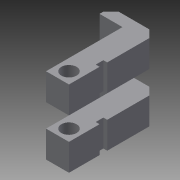
# Autodesk Inventor part: arms01
Saved by Autodesk Inventor 2015 (Build 190159000, 159)
## iProperties
Created: 2016-09-16
Part Number: arms01
Material: Generic
Document SubType Name: Modeling
Designer: spichelh
Density: 1 g/cm^3
Appearance: Default
Author: spichelh
Autodesk Inventor part; units mm, degrees
ref_plane "YZ Plane" through (0, 0, 0) normal (1, 0, 0) x (0, 1, 0)
ref_plane "XZ Plane" through (0, 0, 0) normal (0, 1, 0) x (-1, 0, 0)
ref_plane "XY Plane" through (0, 0, 0) normal (0, 0, 1) x (1, 0, 0)
sketch "Sketch1" plane through (0, 0, 0) normal (0, 0, 1) x (1, 0, 0)
  line L0 (16.7529, 22.7773) -> (28.7529, 22.7773)
  line L1 (28.7529, 22.7773) -> (28.7529, 15.7773)
  line L2 (28.7529, 15.7773) -> (16.7529, 15.7773)
  line L3 (16.7529, 15.7773) -> (16.7529, 22.7773)
  line L4 (16.7529, 9.7773) -> (28.7529, 9.7773)
  line L5 (28.7529, 9.7773) -> (28.7529, 2.7773)
  line L6 (28.7529, 2.7773) -> (16.7529, 2.7773)
  line L7 (16.7529, 2.7773) -> (16.7529, 9.7773)
  point P0 (0, 0)
  dimension "d0" = 7
  dimension "d1" = 6
  dimension "d2" = 12
  constraints: 16 end point, 4 parallel, 2 collinear, 2 horizontal, 2 perpendicular, 1 point on line
  measures "d0" distance of L6.end L4.start
  measures "d1" distance between parallel lines of L2 L4
  measures "d2" distance between parallel lines of L1 L3
extrude "Extrusion1" add sketch "Sketch1" along normal blind 3
sketch "Sketch2" plane through (0, 0, 3) normal (0, 0, 1) x (1, 0, 0)
  line L0 (16.7529, 15.7773) -> (28.7529, 15.7773) projected
  line L1 (28.7529, 22.7773) -> (22.7529, 22.7773)
  line L2 (22.7529, 22.7773) -> (22.7529, 15.7773)
  line L3 (22.7529, 15.7773) -> (28.7529, 15.7773)
  line L4 (28.7529, 15.7773) -> (28.7529, 22.7773)
  line L5 (28.7529, 22.7773) -> (16.7529, 22.7773) projected
  line L6 (28.7529, 15.7773) -> (28.7529, 22.7773) projected
  line L7 (28.7529, 9.7773) -> (22.7529, 9.7773)
  line L8 (22.7529, 9.7773) -> (22.7529, 2.7773)
  line L9 (22.7529, 2.7773) -> (28.7529, 2.7773)
  line L10 (28.7529, 2.7773) -> (28.7529, 9.7773)
  line L11 (16.7529, 2.7773) -> (28.7529, 2.7773) projected
  point P0 (0, 0)
  dimension "d5" = 6
  constraints: 16 end point, 5 parallel, 3 collinear, 2 horizontal, 2 perpendicular, 1 midpoint
  measures "d5" distance between parallel lines of L2 L4
extrude "Extrusion2" add sketch "Sketch2" along normal blind 20
sketch "Sketch3" plane through (16.7529, 22.7773, 0) normal (0, 1, 0) x (1, 0, 0)
  circle A0 centre (9, -20) radius 2
  line L0 (12, -23) -> (6, -23) projected
  line L1 (12, 0) -> (12, -23) projected
  point P0 (-16.7529, 0)
  dimension "d8" = 3
  dimension "d9" = 3
  dimension "d10" = 4
  constraints: 1 centre point
  measures "d8" distance from line of L0 A0.centre
  measures "d9" distance from line of L1 A0.centre
  measures "d10" diameter of A0
extrude "Extrusion3" cut sketch "Sketch3" against normal blind 30
chamfer "Chamfer1" distance 2 angle 45 4 edges at (28.7529, 19.2773, 0) (16.7529, 19.2773, 0) (28.7529, 6.2773, 0) (16.7529, 6.2773, 0)
sketch "Sketch4" plane through (28.7529, 15.7773, 23) normal (1, 0, 0) x (0, 0, -1)
  line L0 (8, 11.5882) -> (10, 11.5882)
  line L1 (10, 11.5882) -> (10, -21.6618)
  line L2 (10, -21.6618) -> (8, -21.6618)
  line L3 (8, -21.6618) -> (8, 11.5882)
  line L4 (0, 0) -> (0, 7) projected
  point P0 (23, -15.7773)
  dimension "d16" = 2
  dimension "d17" = 8
  constraints: 8 end point, 2 parallel, 1 horizontal, 1 perpendicular
  measures "d16" distance between parallel lines of L3 L1
  measures "d17" distance between parallel lines of L4 L3
extrude "Extrusion4" cut sketch "Sketch4" against normal blind 1
body "Solid1"
